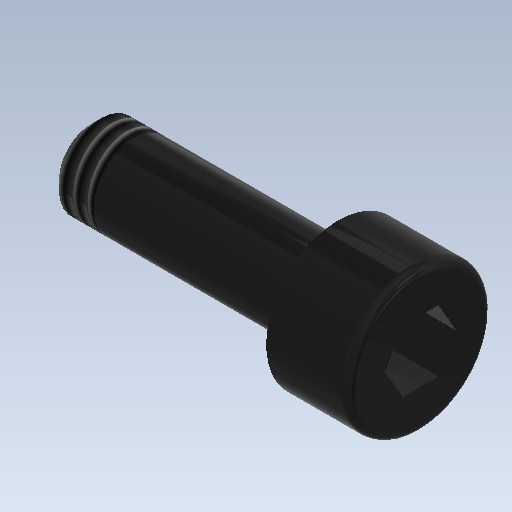
# Autodesk Inventor part: Slotted head cap screw ISO 4762 - M4x12
Saved by Autodesk Inventor 2021 (Build 250183000, 183)
## iProperties
Category: PARTsolutions
Company: MISUMI
Part Number: Slotted head cap screw ISO 4762 - M4x12
Material: ステンレス鋼
Catalog Web Link: www.cadenas.de
Description: ISO 4762-Hexagon socket head cap screw
Vendor: MISUMI
Document SubType Name: Modeling
Designer: partserver
Manufacturer: MISUMI
Mass: 2.25154 g
Surface Area: 3.34196 cm^2
Volume: 0.281442 cm^3
Density: 8 g/cm^3
Appearance: 滑らか - 黒
PSOL_IDENT_0: {$CADENAS_DATA\23d-libs\misumi\metric\accessories\din_en_iso_4762.prj},223 {VTYP=3D},{NB=Slotted hea
PSOL_IDENT_1: d cap screw ISO 4762 - M4x12},{LINA=Slotted head cap screw ISO 4762 - M4x12},{NN=ISO 4762},{DATE=12.
PSOL_IDENT_2: 12.2019 00:47:08},{GEOMDATE=17.02.2014 00:00:00},{VERSION=v1},{LINEID=400},{WBVAR=},{WBNUMERIC=}  {N
PSOL_IDENT_3: B=Zylinderschraube ISO 4762 - M4x12},{LINA=Zylinderschraube ISO 4762 - M4x12},{KT=DUMMY},{IDNR=},{D=
PSOL_IDENT_4: 4.000},{D3=3.141},{P=0.700},{L=12.000},{S=3.000},{HM=12.000},{DK=7.000},{DA=4.700},{DS=4.000},{E=3.4
PSOL_IDENT_5: 40},{K=4.000},{R=0.200},{T=2.000},{V=0.400},{DW=6.530},{W=1.400},{LF=0.600},{LG=2.100},{FORM=1.000},
PSOL_IDENT_6: {NENN=M4x12}
NB: Slotted head cap screw ISO 4762 - M4x12
NN: ISO 4762
NT: Hexagon socket head cap screw
NBSYN: Slotted head cap screw ISO 4762 - $NENN.
LINA: Slotted head cap screw ISO 4762 - M4x12
CATALOG: Misumi
ROWDESC: M4x12
D: 4
D3: 3.141
P: 0.7
L: 12
S: 3
HM: 12
DK: 7
DA: 4.7
DS: 4
E: 3.44
K: 4
R: 0.2
T: 2
V: 0.4
DW: 6.53
W: 1.4
LF: 0.6
LG: 2.1
FORM: 1
SUPPLIER: MISUMI
ARTICLENO: Slotted head cap screw ISO 4762 - M4x12
BOMINFO: Slotted head cap screw ISO 4762 - M4x12
CREATOR: CADENAS GmbH
d5: 0.000 mm
d6: 0.000 mm
d7: 0.000 mm
d8: 0.000 mm
Title: Slotted head cap screw ISO 4762 - M4x12
Author: Cadenas PARTsolutions
Comments: Hexagon socket head cap screw
Autodesk Inventor part; units mm, degrees
sketch "Skizze_2" plane through (0, 0, 0) normal (0, 0, 1) x (1, 0, 0)
  line L0 (12, 0) -> (-0.534, 0)
  line L1 (-0.534, 0) -> (-1.4, 1.5)
  line L2 (-1.4, 1.5) -> (-4, 1.5)
  line L3 (-4, 1.5) -> (-4, 3.1)
  arc A0 (-3.6, 3.5) -> (-4, 3.1) centre (-3.6, 3.1) ccw
  line L4 (-3.6, 3.5) -> (0, 3.5)
  line L5 (0, 3.5) -> (0, 2.35)
  arc A1 (0, 2.35) -> (0.1298, 2.1627) centre (0.2, 2.35) ccw
  line L6 (0.1298, 2.1627) -> (0.5298, 2.0127)
  arc A2 (0.5298, 2.0127) -> (0.6, 2) centre (0.6, 2.2) ccw
  line L7 (0.6, 2) -> (11.5705, 2)
  line L8 (11.5705, 2) -> (12, 1.5705)
  line L9 (12, 1.5705) -> (12, 0)
  line L10 (12, 0) -> (-0.534, 0)
  constraints: 22 end point, 6 point on circle, 3 centre point
revolve "Revolution1" add sketch "Skizze_2" angle 360 about axis through (12, 0, 0) along (1, 0, 0)
thread "Thread1" size "M4x0.7" class "6g" standard "ISO Metric profile" length 1.6705
sketch "Skizze_1" plane through (-1.4, 0, 0) normal (1, 0, 0) x (0, 0, -1)
  line L0 (-1.5, -0.866) -> (0, -1.7321)
  line L1 (0, -1.7321) -> (1.5, -0.866)
  line L2 (1.5, -0.866) -> (1.5, 0.866)
  line L3 (1.5, 0.866) -> (0, 1.7321)
  line L4 (0, 1.7321) -> (-1.5, 0.866)
  line L5 (-1.5, 0.866) -> (-1.5, -0.866)
  constraints: 12 end point
extrude "Extrusion1" cut sketch "Skizze_1" against normal blind 4
ref_plane "IP1_XY" through (0, 0, 0) normal (1, 0, 0) x (0, 0, -1)
ref_plane "IP1_YZ" through (0, 0, 0) normal (0, 0, -1) x (0, 1, 0)
ref_plane "IP1_ZX" through (0, 0, 0) normal (0, 1, 0) x (1, 0, 0)
ref_plane "IP2_XY" through (-4, 0, 0) normal (1, 0, 0) x (0, 0, -1)
ref_plane "IP2_YZ" through (-4, 0, 0) normal (0, 0, -1) x (0, 1, 0)
ref_plane "IP2_ZX" through (-4, 0, 0) normal (0, 1, 0) x (1, 0, 0)
ref_plane "IP3_XY" through (12, 0, 0) normal (1, 0, 0) x (0, 0, -1)
ref_plane "IP3_YZ" through (12, 0, 0) normal (0, 0, -1) x (0, 1, 0)
ref_plane "IP3_ZX" through (12, 0, 0) normal (0, 1, 0) x (1, 0, 0)
ref_plane "IP4_XY" through (0, 0, 0) normal (1, 0, 0) x (0, 0, -1)
ref_plane "IP4_YZ" through (0, 0, 0) normal (0, 0, -1) x (0, 1, 0)
ref_plane "IP4_ZX" through (0, 0, 0) normal (0, 1, 0) x (1, 0, 0)
body "Solid1"
